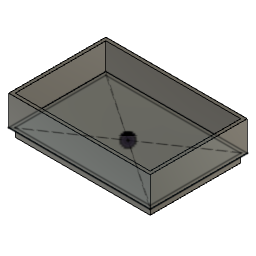
Container v2 (Autodesk Fusion 360 design; units mm, degrees)
Autodesk Fusion 360 part; units mm, degrees
sketch "Sketch1" plane through (0, 0, 0) normal (0, 0, 1) x (1, 0, 0)
  line L0 (-63.395, 42.575) -> (63.395, 42.575)
  line L1 (63.395, 42.575) -> (63.395, -42.575)
  line L2 (63.395, -42.575) -> (-63.395, -42.575)
  line L3 (-63.395, -42.575) -> (-63.395, 42.575)
  line L4 (-63.395, 42.575) -> (63.395, -42.575) construction
  line L5 (63.395, 42.575) -> (-63.395, -42.575) construction
  dimension "d1" = 126.79
  dimension "d2" = 85.15
  constraint horizontal L0
  constraint perpendicular L0 L1
  constraint parallel L0 L2
  constraint parallel L1 L3
  constraint coincident L4 origin
  constraint coincident L5 origin
  measures "d1" distance of L1.end L2.end
  measures "d2" distance of L0.end L1.end
sketch "Sketch2" plane through (0, 0, 0) normal (0, 1, 0) x (1, 0, 0)
sketch "Sketch3" plane through (0, 0, 0) normal (0, 0, 1) x (1, 0, 0)
  line L0 (66.395, -45.575) -> (-66.395, -45.575)
  line L1 (-66.395, -45.575) -> (-66.395, 45.575)
  line L2 (-66.395, 45.575) -> (66.395, 45.575)
  line L3 (66.395, 45.575) -> (66.395, -45.575)
  line L4 (66.395, -45.575) -> (-66.395, 45.575) construction
  line L5 (-66.395, -45.575) -> (66.395, 45.575) construction
  dimension "d3" = 132.79
  dimension "d4" = 91.15
  constraint horizontal L0
  constraint perpendicular L0 L1
  constraint parallel L0 L2
  constraint parallel L1 L3
  constraint coincident L4 origin
  constraint coincident L5 origin
  measures "d3" distance of L1.end L2.end
  measures "d4" distance of L0.end L1.end
extrude "Extrude1" add sketch "Sketch3" along normal blind 28
shell "Shell1" thickness 3 removed faces 1 at (-22.1317, 15.1917, 28)
extrude "Extrude2" add sketch "Sketch1" against normal blind 4
extrude "Extrude3" add 1 faces at (-21.1317, 14.1917, -4) along direction (0, 0, -1) blind 3.9
